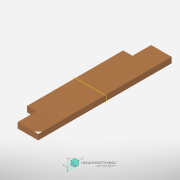
# Autodesk Inventor part: MPX-rib
Saved by Autodesk Inventor 2016 (Build 200138000, 138)
## iProperties
Created: 2015-05-27
Part Number: MPX-rib
Material: Wood (Cherry)
Document SubType Name: Modeling
Designer: as
Mass: 247.023 g
Surface Area: 654.2 cm^2
Volume: 392.1 cm^3
Density: 0.63 g/cm^3
Appearance: Cherry - Natural Low Gloss
Author: as
Autodesk Inventor part; units mm, degrees
ref_plane "YZ Plane" through (0, 0, 0) normal (1, 0, 0) x (0, 1, 0)
ref_plane "XZ Plane" through (0, 0, 0) normal (0, 1, 0) x (-1, 0, 0)
ref_plane "XY Plane" through (0, 0, 0) normal (0, 0, 1) x (1, 0, 0)
sketch "Sketch1" plane through (0, 0, 0) normal (0, 0, 1) x (1, 0, 0)
  line L0 (0, 0) -> (-80, 0)
  line L1 (-80, 0) -> (-80, 358)
  line L2 (-80, 358) -> (0, 358)
  line L3 (0, 358) -> (0, 0)
  dimension "d0" = 80
  dimension "d1" = 358
  constraints: 8 end point, 2 parallel, 1 horizontal, 1 perpendicular
  measures "d0" distance of L1.end L2.end
  measures "d1" distance of L0.end L1.end
extrude "Extrusion1" add sketch "Sketch1" along normal blind 15
sketch "Sketch2" plane through (0, 0, 15) normal (0, 0, 1) x (1, 0, 0)
  line L0 (-80, 0) -> (0, 0) projected
  line L1 (-80, 0) -> (-55, 0)
  line L2 (-55, 0) -> (-55, 50)
  line L3 (-55, 50) -> (-80, 50)
  line L4 (-80, 50) -> (-80, 0)
  dimension "d4" = 25
  dimension "d5" = 50
  constraints: 8 end point, 2 parallel, 1 horizontal, 1 perpendicular
  measures "d4" distance of L3.end L2.end
  measures "d5" distance of L2.end L1.end
extrude "Extrusion2" cut sketch "Sketch2" against normal through all
ref_plane "Work Plane1" through (0, 179, 0) normal (0, -1, 0) x (1, 0, 0)
mirror "Mirror1" about plane through (0, 179, 0) normal (0, -1, 0) of "Extrusion2"
body "Solid1"
